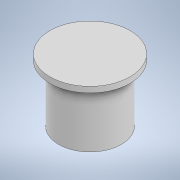
# Autodesk Inventor part: tulejapodstawa
Saved by Autodesk Inventor 2022 (Build 260153000, 153)
## iProperties
Created: 2022-03-29
Part Number: tulejapodstawa
Material: Ogólny
Document SubType Name: Modeling
Designer: jolow
Density: 1 g/cm^3
Appearance: Domyślna
Author: jolow
Autodesk Inventor part; units mm, degrees
ref_plane "YZ Plane" through (0, 0, 0) normal (1, 0, 0) x (0, 1, 0)
ref_plane "XZ Plane" through (0, 0, 0) normal (0, 1, 0) x (-1, 0, 0)
ref_plane "XY Plane" through (0, 0, 0) normal (0, 0, 1) x (1, 0, 0)
sketch "Szkic1" plane through (0, 0, 0) normal (0, 1, 0) x (-1, 0, 0)
  circle A0 centre (0, 0) radius 11
  circle A1 centre (0, 0) radius 9
  dimension "d0" = 22
  dimension "d1" = 2
  constraints: 2 centre point, 2 coincident
  measures "d0" diameter of A0
  measures "d1" radial gap between concentric circles of A0 A1
extrude "Wyciągnięcie proste1" add sketch "Szkic1" along normal blind 20
sketch "Szkic2" plane through (0, 20, 0) normal (0, 1, 0) x (1, 0, 0)
  circle A0 centre (0, 0) radius 14
  circle A1 centre (0, 0) radius 11 projected
  dimension "d4" = 28
  dimension "d7" = 3
  constraints: 1 centre point, 1 coincident
  measures "d4" diameter of A0
  measures "d7" radial gap between concentric circles of A1 A0
extrude "Wyciągnięcie proste2" add sketch "Szkic2" along normal blind 2 contours A0 | A1
